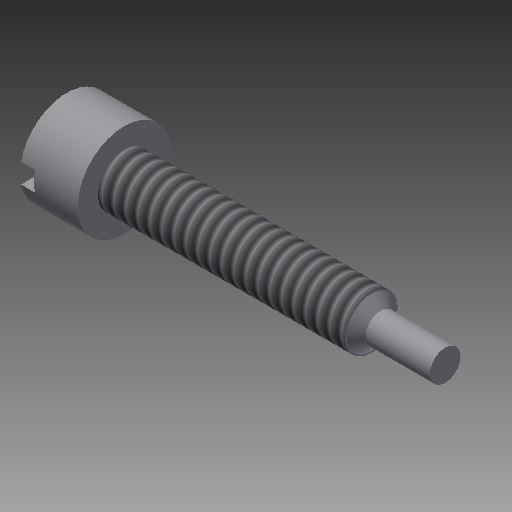
# Autodesk Inventor part: Air Adjuster
Saved by Autodesk Inventor 2017 (Build 210135000, 135)
## iProperties
Created: 2012-08-08
Part Number: Air Adjuster
Material: Generic
Document SubType Name: Modeling
Designer: John
Density: 1 g/cm^3
Appearance: Default
Author: John
Autodesk Inventor part; units mm, degrees
ref_plane "YZ Plane" through (0, 0, 0) normal (1, 0, 0) x (0, 1, 0)
ref_plane "XZ Plane" through (0, 0, 0) normal (0, 1, 0) x (-1, 0, 0)
ref_plane "XY Plane" through (0, 0, 0) normal (0, 0, 1) x (1, 0, 0)
sketch "Sketch1" plane through (0, 0, 0) normal (1, 0, 0) x (0, 1, 0)
  circle A0 centre (0, 0) radius 2.4765
  dimension "d1" = 4.953
  constraints: 1 centre point, 1 coincident
  measures "d1" diameter of A0
extrude "Extrusion1" add sketch "Sketch1" along normal blind 3.048
sketch "Sketch2" plane through (3.048, 0, 0) normal (1, 0, 0) x (0, 0, -1)
  circle A0 centre (0, 0) radius 2.4765 projected
  circle A1 centre (0, 0) radius 1.397
  dimension "d5" = 2.794
  constraints: 1 centre point, 1 coincident
  measures "d5" diameter of A1
extrude "Extrusion2" add sketch "Sketch2" along normal blind 13.081 contours A1
sketch "Sketch3" plane through (16.129, 0, 0) normal (1, 0, 0) x (0, 0, -1)
  circle A0 centre (0, 0) radius 1.397 projected
  circle A1 centre (0, 0) radius 0.8128
  dimension "d8" = 1.6256
  constraints: 1 centre point, 1 coincident
  measures "d8" diameter of A1
extrude "Extrusion3" add sketch "Sketch3" along normal blind 3.9116 contours A1
chamfer "Chamfer1" distance 0.508 angle 45 1 edges at (16.129, 0, 0.8128)
thread "Thread1" size "4-40 UNC" class "2A" standard "ANSI Unified Screw Threads" full length
sketch "Sketch4" plane through (0, 0, 0) normal (-1, 0, 0) x (0, 0, 1)
  circle A0 centre (0, 0) radius 2.4765 projected
  line L0 (-2.4765, 0.5207) -> (2.4765, 0.5207)
  line L1 (2.4765, 0.5207) -> (2.4765, -0.5207)
  line L2 (2.4765, -0.5207) -> (-2.4765, -0.5207)
  line L3 (-2.4765, -0.5207) -> (-2.4765, 0.5207)
  dimension "d16" = 1.0414
  dimension "d18" = 0.5207
  constraints: 8 end point, 2 parallel, 2 tangent, 1 horizontal, 1 perpendicular
  measures "d16" distance of L0.end L1.end
  measures "d18" distance from line of A0.centre L2
extrude "Extrusion4" cut sketch "Sketch4" against normal blind 0.7366 contours A0 L2 L0 | L1 L2 A0 | A0 L0 L1 | A0 L3 L0 | L2 L3 A0
equation "\"d18\" = 0.5 * d16"
body "Solid1"
